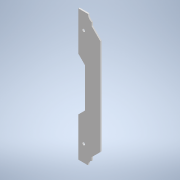
# Autodesk Inventor part: domePlace
Saved by Autodesk Inventor 2022 (Build 260153000, 153)
## iProperties
Created: 2021-07-01
Part Number: domePlace
Material: Generic
Document SubType Name: Modeling
Designer: dsdan
Density: 1 g/cm^3
Appearance: Default
Author: dsdan
Autodesk Inventor part; units mm, degrees
ref_plane "YZ Plane" through (0, 0, 0) normal (1, 0, 0) x (0, 1, 0)
ref_plane "XZ Plane" through (0, 0, 0) normal (0, 1, 0) x (-1, 0, 0)
ref_plane "XY Plane" through (0, 0, 0) normal (0, 0, 1) x (1, 0, 0)
sketch "Sketch1" plane through (0, 0, 0) normal (0, 0, 1) x (1, 0, 0)
  circle A0 centre (0, 0) radius 12.5
  circle A1 centre (0, -298.822) radius 12.5
  line L0 (-114.8008, 0.589) -> (-4.5, 0.589)
  line L1 (-4.5, 0.589) -> (-4.5, -299.411)
  line L2 (-4.5, -299.411) -> (-114.8008, -299.411)
  line L3 (-114.8008, -299.411) -> (-114.8008, 0.589) construction
  line L4 (-114.8008, 0.589) -> (-4.5, -299.411) construction
  line L5 (-4.5, 0.589) -> (-114.8008, -299.411) construction
  line L6 (-114.8008, -2.4111) -> (-114.8008, -296.4111) construction
  line L7 (-4.5, -19.411) -> (15.5, -39.411)
  line L8 (15.5, -39.411) -> (15.5, -259.411)
  line L9 (15.5, -259.411) -> (-4.5, -279.411)
  line L10 (-34.5, 0.589) -> (-34.5, -89.411)
  line L11 (-34.5, -89.411) -> (-19.5, -104.411)
  line L12 (-19.5, -104.411) -> (-19.5, -194.411)
  line L13 (-19.5, -194.411) -> (-34.5, -209.411)
  line L14 (-34.5, -209.411) -> (-34.5, -299.411)
  circle A2 centre (-22.6008, -36.9111) radius 3.5 construction
  circle A3 centre (-22.6008, -261.9111) radius 3.5 construction
  circle A4 centre (-22.6008, -36.9111) radius 3
  circle A5 centre (-22.6008, -261.9111) radius 3
  point P0 (-59.6504, -149.411)
  point P1 (12.4861, 0.589)
  point P2 (-12.4861, 0.589)
  point P3 (-12.4861, -299.411)
  point P4 (12.4861, -299.411)
  point P5 (-4.5, -287.1601)
  point P6 (-4.5, -11.6619)
  dimension "d0" = 25
  dimension "d1" = 25
  dimension "d2" = 298.822
  dimension "d3" = 300
  dimension "d4" = 149.411
  dimension "d6" = 149.411
  dimension "d9" = 4.5
  dimension "d10" = 45
  dimension "d11" = 45
  dimension "d12" = 20
  dimension "d13" = 20
  dimension "d14" = 20
  dimension "d15" = 45
  dimension "d16" = 45
  dimension "d17" = 90
  dimension "d18" = 90
  dimension "d19" = 30
  dimension "d20" = 90
  dimension "d21" = 6
  dimension "d22" = 6
  constraints: 28 end point, 6 point on line, 4 centre point, 3 coincident, 3 vertical, 2 midpoint, 2 parallel, 1 collinear, 1 horizontal, 1 perpendicular, 1 vertical alignment
  measures "d0" diameter of A0
  measures "d1" diameter of A1
  measures "d2" distance of A1.centre A0.centre
  measures "d3" distance between parallel lines of L0 L2
  measures "d4" vertical distance of A0.centre point (-59.65, -149.411)
  measures "d6" vertical distance of A1.centre point (-59.65, -149.411)
  measures "d9" distance from line of A0.centre L1
  measures "d10" angle of L1 L7
  measures "d11" angle of L1 L9
  measures "d12" distance from line of L0 L7.start
  measures "d13" distance from line of L2 L9.end
  measures "d14" distance between parallel lines of L1 L8
  measures "d15" angle of L10 L11
  measures "d16" angle of L14 L13
  measures "d17" distance of L10.start L10.end
  measures "d18" distance of L13.end L14.end
  measures "d19" distance between parallel lines of L1 L10
  measures "d20" distance of L11.end L12.end
  measures "d21" diameter of A4
  measures "d22" diameter of A5
extrude "Extrusion1" add sketch "Sketch1" along normal blind 3 contours A0 L1 A1 L2 L14 L13 L12 L11 L10 L0 | L7 L8 L9 L1
equation "\"d4\" = d6"
body "Solid1"
